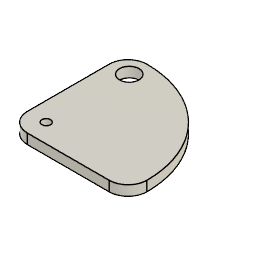
smartie_arm (Autodesk Fusion 360 design; units mm, degrees)
Autodesk Fusion 360 part; units mm, degrees
sketch "Smartie arm" plane through (0, 0, 0) normal (0, 0, 1) x (1, 0, 0)
  line L0 (0, 0) -> (95, 0)
  line L1 (95, 0) -> (95, 95)
  line L2 (95, 95) -> (0, 95)
  line L3 (0, 95) -> (0, 0)
  dimension "d6" = 95
  dimension "d15" = 95
  constraint horizontal L0
  constraint vertical L1
  constraint horizontal L2
  constraint vertical L3
  constraint coincident L0.start L3.end
  measures "d6" distance of L1.end L2.end
  measures "d15" distance of L0.end L1.end
extrude "Extrude1" add sketch "Smartie arm" along normal blind 8
sketch "Smartie hole" plane through (0, 0, 8) normal (0, 0, 1) x (-1, 0, 0)
  line L0 (0, -95) -> (0, 0)
  line L1 (0, 0) -> (-95, 0)
  line L2 (-95, 0) -> (-95, -95)
  line L3 (-95, -95) -> (0, -95)
  circle A0 centre (-15, -81) radius 7.75
  dimension "d5" = 15.5
  dimension "d8" = 15
  dimension "d9" = 80
  dimension "d14" = 14
  measures "d5" diameter of A0
  measures "d8" distance of L0 A0.centre
  measures "d9" distance of L2 A0.centre
  measures "d14" distance of L3 A0.centre
extrude "Extrude2" cut sketch "Smartie hole" against normal blind 8 contours A0
fillet "Fillet1" radius 15 2 edges at (95, 95, 4) (0, 95, 4)
fillet "Fillet2" radius 15 2 edges at (0, 0, 4) (95, 0, 4)
sketch "Smartie arm arc" plane through (0, 0, 8) normal (0, 0, 1) x (-1, 0, 0)
  arc A0 (-80, 0) -> (-95, -15) centre (-80, -15) ccw
  line L0 (-95, -15) -> (-95, -80)
  arc A1 (-95, -80) -> (-80, -95) centre (-80, -80) ccw
  line L1 (-80, -95) -> (-15, -95)
  arc A2 (-15, -95) -> (0, -80) centre (-15, -80) ccw
  line L2 (0, -80) -> (0, -15)
  arc A3 (0, -15) -> (-15, 0) centre (-15, -15) ccw
  line L3 (-15, 0) -> (-80, 0)
  circle A4 centre (-15, -81) radius 7.75
  circle A5 centre (-15, -15) radius 80
  dimension "d16" = 15
  dimension "d17" = 15
  dimension "d18" = 160
  measures "d16" horizontal distance of L2.end A3.centre
  measures "d17" distance of L3 A3.centre
  measures "d18" diameter of A5
extrude "Extrude3" cut sketch "Smartie arm arc" against normal blind 8 contours L0 A1 L1 A5
sketch "Servo horn hole" plane through (0, 0, 0) normal (0, 0, -1) x (1, 0, 0)
  arc A0 (15, -95) -> (95, -15) centre (15, -15) ccw
  arc A1 (95, -15) -> (80, 0) centre (80, -15) ccw
  line L0 (80, 0) -> (15, 0)
  arc A2 (15, 0) -> (0, -15) centre (15, -15) ccw
  line L1 (0, -15) -> (0, -80)
  arc A3 (0, -80) -> (15, -95) centre (15, -80) ccw
  circle A4 centre (15, -81) radius 7.75
  circle A5 centre (15, -15) radius 10.25
  circle A6 centre (15, -15) radius 3.5
  dimension "d21" = 20.5
  dimension "d24" = 7
  constraint concentric A0 A5
  constraint concentric A5 A6
  measures "d21" diameter of A5
  measures "d24" diameter of A6
extrude "Extrude4" cut sketch "Servo horn hole" against normal blind 1.2 contours A5 | A6
extrude "Extrude5" cut sketch "Servo horn hole" against normal blind 8 contours A6
equation "d14 = 16 mm - 2 mm"
named bodies: "Smartie arm"
